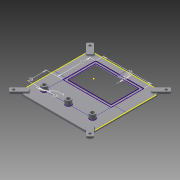
# Autodesk Inventor part: LX4000 2x3slide holder
Saved by Autodesk Inventor 2013 SP2 (Build 170200200, 200)
## iProperties
Created: 2015-05-08
Part Number: LX4000 2x3slide holder
Material: Generic
Document SubType Name: Modeling
Designer: kthorn
Density: 1 g/cm^3
Author: kthorn
Autodesk Inventor part; units mm, degrees
ref_plane "YZ Plane" through (0, 0, 0) normal (1, 0, 0) x (0, 1, 0)
ref_plane "XZ Plane" through (0, 0, 0) normal (0, 1, 0) x (-1, 0, 0)
ref_plane "XY Plane" through (0, 0, 0) normal (0, 0, 1) x (1, 0, 0)
sketch "Sketch1" plane through (0, 0, 0) normal (0, 0, 1) x (1, 0, 0)
  line L0 (-34.939227, 36.850829) -> (65.060773, 36.850829)
  line L1 (73.060773, 28.850829) -> (73.060773, -71.149171)
  line L2 (65.060773, -79.149171) -> (-34.939227, -79.149171)
  line L3 (-42.939227, -71.149171) -> (-42.939227, 28.850829)
  arc A0 (-34.939227, 36.850829) -> (-42.939227, 28.850829) centre (-34.939227, 28.850829) ccw
  arc A1 (-42.939227, -71.149171) -> (-34.939227, -79.149171) centre (-34.939227, -71.149171) ccw
  arc A2 (65.060773, -79.149171) -> (73.060773, -71.149171) centre (65.060773, -71.149171) ccw
  arc A3 (73.060773, 28.850829) -> (65.060773, 36.850829) centre (65.060773, 28.850829) ccw
  point P0 (0, 0)
  point P1 (-42.939227, 36.850829)
  point P2 (73.060773, 36.850829)
  dimension "d0" = 116
  dimension "d2" = 8
  constraints: 8 end point, 8 point on circle, 8 tangent, 4 centre point, 4 point on line, 3 equal radius, 2 parallel, 2 perpendicular, 1 horizontal
  measures "d0" distance of point (-42.939, 36.851) point (73.061, 36.851)
  measures "d2" radius of A0
extrude "Extrusion1" add sketch "Sketch1" along normal blind 3.1
sketch "Sketch2" plane through (0, 0, 3.1) normal (0, 0, 1) x (1, 0, 0)
  line L0 (-42.939227, 28.850829) -> (-42.939227, -71.149171)
  line L1 (73.060773, -71.149171) -> (73.060773, 28.850829)
  line L2 (65.060773, 36.850829) -> (-34.939227, 36.850829)
  line L3 (-23.939227, 26.850829) -> (54.060773, 26.850829)
  line L4 (54.060773, 26.850829) -> (54.060773, -26.149171)
  line L5 (54.060773, -26.149171) -> (-23.939227, -26.149171)
  line L6 (-23.939227, -26.149171) -> (-23.939227, 26.850829)
  line L7 (-19.939227, 22.850829) -> (50.060773, 22.850829)
  line L8 (50.060773, 22.850829) -> (50.060773, -22.149171)
  line L9 (50.060773, -22.149171) -> (-19.939227, -22.149171)
  line L10 (-19.939227, -22.149171) -> (-19.939227, 22.850829)
  line L11 (15.060773, -26.149171) -> (15.060773, -22.149171) construction
  line L12 (-23.939227, 0.350829) -> (-19.939227, 0.350829) construction
  line L13 (15.060773, 26.850829) -> (15.060773, 22.850829) construction
  line L14 (50.060773, 0.350829) -> (54.060773, 0.350829) construction
  line L15 (-23.939227, -21.149171) -> (-42.939227, -21.149171) construction
  line L16 (54.060773, -21.149171) -> (73.060773, -21.149171) construction
  line L17 (15.060773, 36.850829) -> (15.060773, 26.850829) construction
  dimension "d5" = 78
  dimension "d7" = 53
  dimension "d8" = 4
  dimension "d23" = 10
  constraints: 30 end point, 12 midpoint, 8 perpendicular, 4 equal length, 4 parallel, 2 horizontal, 2 point on line, 1 vertical
  measures "d5" distance of L3.start L3.end
  measures "d7" distance of L5.end L3.start
  measures "d8" distance of L13.start L13.end
  measures "d23" distance of L17.start L17.end
extrude "Extrusion2" cut sketch "Sketch2" against normal up to next contours L7 L8 L9 L10
extrude "Extrusion3" cut sketch "Sketch2" against normal blind 1.5
sketch "Sketch3" plane through (0, 0, 3.1) normal (0, 0, 1) x (1, 0, 0)
  line L0 (-34.939227, -79.149171) -> (65.060773, -79.149171)
  line L1 (65.060773, 36.850829) -> (-34.939227, 36.850829)
  line L2 (-42.939227, -71.149171) -> (-42.939227, -79.149171) construction
  line L3 (-34.939227, -79.149171) -> (-42.939227, -79.149171) construction
  line L4 (-42.939227, -79.149171) -> (-42.939227, -82.899171) construction
  line L5 (-42.939227, -82.899171) -> (-46.689227, -82.899171) construction
  line L6 (-32.658004, -75.231909) -> (-46.093032, -88.666938)
  line L7 (-48.92146, -88.666938) -> (-52.456993, -85.131404)
  line L8 (-52.456993, -82.302977) -> (-39.021965, -68.867948)
  line L9 (-36.193538, -68.867948) -> (-32.658004, -72.403482)
  line L10 (-46.689227, -82.899171) -> (-46.689227, -86.899171) construction
  line L11 (-46.689227, -86.899171) -> (-50.689227, -86.899171) construction
  circle A0 centre (-46.689227, -82.899171) radius 2
  arc A1 (-52.456993, -82.302977) -> (-52.456993, -85.131404) centre (-51.04278, -83.71719) ccw
  arc A2 (-48.92146, -88.666938) -> (-46.093032, -88.666938) centre (-47.507246, -87.252724) ccw
  arc A3 (-36.193538, -68.867948) -> (-39.021965, -68.867948) centre (-37.607751, -70.282162) ccw
  arc A4 (-32.658004, -75.231909) -> (-32.658004, -72.403482) centre (-34.072217, -73.817696) ccw
  line L12 (-23.939227, -26.149171) -> (-23.939227, 26.850829)
  line L13 (-23.939227, 26.850829) -> (54.060773, 26.850829)
  line L14 (54.060773, 26.850829) -> (54.060773, -26.149171)
  line L15 (54.060773, -26.149171) -> (-23.939227, -26.149171)
  line L16 (-42.939227, 28.850829) -> (-42.939227, -71.149171)
  arc A5 (-42.939227, -71.149171) -> (-34.939227, -79.149171) centre (-34.939227, -71.149171) ccw
  line L17 (-34.939227, -79.149171) -> (65.060773, -79.149171)
  arc A6 (65.060773, -79.149171) -> (73.060773, -71.149171) centre (65.060773, -71.149171) ccw
  line L18 (73.060773, -71.149171) -> (73.060773, 28.850829)
  arc A7 (73.060773, 28.850829) -> (65.060773, 36.850829) centre (65.060773, 28.850829) ccw
  line L19 (65.060773, 36.850829) -> (-34.939227, 36.850829)
  arc A8 (-34.939227, 36.850829) -> (-42.939227, 28.850829) centre (-34.939227, 28.850829) ccw
  line L20 (15.060773, -79.149171) -> (15.060773, 36.850829) construction
  line L21 (73.060773, -21.149171) -> (-42.939227, -21.149171) construction
  line L22 (73.060773, -71.149171) -> (73.060773, -79.149171) construction
  line L23 (65.060773, -79.149171) -> (73.060773, -79.149171) construction
  line L24 (73.060773, -79.149171) -> (73.060773, -82.899171) construction
  line L25 (73.060773, -82.899171) -> (76.810773, -82.899171) construction
  line L26 (62.779551, -75.231909) -> (76.214579, -88.666938)
  line L27 (79.043007, -88.666938) -> (82.57854, -85.131404)
  line L28 (82.57854, -82.302977) -> (69.143512, -68.867948)
  line L29 (66.315084, -68.867948) -> (62.779551, -72.403482)
  line L30 (76.810773, -82.899171) -> (76.810773, -86.899171) construction
  line L31 (76.810773, -86.899171) -> (80.810773, -86.899171) construction
  circle A9 centre (76.810773, -82.899171) radius 2
  arc A10 (82.57854, -85.131404) -> (82.57854, -82.302977) centre (81.164327, -83.71719) ccw
  arc A11 (76.214579, -88.666938) -> (79.043007, -88.666938) centre (77.628793, -87.252724) ccw
  arc A12 (69.143512, -68.867948) -> (66.315084, -68.867948) centre (67.729298, -70.282162) ccw
  arc A13 (62.779551, -72.403482) -> (62.779551, -75.231909) centre (64.193764, -73.817696) ccw
  arc A14 (65.060773, -79.149171) -> (73.060773, -71.149171) centre (65.060773, -71.149171) ccw
  line L32 (-42.939227, 28.850829) -> (-42.939227, 36.850829) construction
  line L33 (-34.939227, 36.850829) -> (-42.939227, 36.850829) construction
  line L34 (-42.939227, 36.850829) -> (-42.939227, 40.600829) construction
  line L35 (-42.939227, 40.600829) -> (-46.689227, 40.600829) construction
  line L36 (-32.658004, 32.933567) -> (-46.093032, 46.368596)
  line L37 (-48.92146, 46.368596) -> (-52.456993, 42.833062)
  line L38 (-52.456993, 40.004635) -> (-39.021965, 26.569606)
  line L39 (-36.193538, 26.569606) -> (-32.658004, 30.10514)
  line L40 (-46.689227, 40.600829) -> (-46.689227, 44.600829) construction
  line L41 (-46.689227, 44.600829) -> (-50.689227, 44.600829) construction
  circle A15 centre (-46.689227, 40.600829) radius 2
  arc A16 (-52.456993, 42.833062) -> (-52.456993, 40.004635) centre (-51.04278, 41.418849) ccw
  arc A17 (-46.093032, 46.368596) -> (-48.92146, 46.368596) centre (-47.507246, 44.954382) ccw
  arc A18 (-39.021965, 26.569606) -> (-36.193538, 26.569606) centre (-37.607751, 27.98382) ccw
  arc A19 (-32.658004, 30.10514) -> (-32.658004, 32.933567) centre (-34.072217, 31.519354) ccw
  arc A20 (-34.939227, 36.850829) -> (-42.939227, 28.850829) centre (-34.939227, 28.850829) ccw
  arc A21 (73.060773, 28.850829) -> (65.060773, 36.850829) centre (65.060773, 28.850829) ccw
  arc A22 (62.779551, 32.933567) -> (62.779551, 30.10514) centre (64.193764, 31.519354) ccw
  line L42 (66.315084, 26.569606) -> (62.779551, 30.10514)
  arc A23 (66.315084, 26.569606) -> (69.143512, 26.569606) centre (67.729298, 27.98382) ccw
  arc A24 (73.060773, 28.850829) -> (65.060773, 36.850829) centre (65.060773, 28.850829) ccw
  line L43 (73.060773, 28.850829) -> (73.060773, 36.850829) construction
  line L44 (65.060773, 36.850829) -> (73.060773, 36.850829) construction
  line L45 (73.060773, 36.850829) -> (73.060773, 40.600829) construction
  line L46 (73.060773, 40.600829) -> (76.810773, 40.600829) construction
  line L47 (62.779551, 32.933567) -> (76.214579, 46.368596)
  line L48 (79.043007, 46.368596) -> (82.57854, 42.833062)
  line L49 (82.57854, 40.004635) -> (69.143512, 26.569606)
  line L50 (76.810773, 40.600829) -> (76.810773, 44.600829) construction
  line L51 (76.810773, 44.600829) -> (80.810773, 44.600829) construction
  circle A25 centre (76.810773, 40.600829) radius 2
  arc A26 (82.57854, 40.004635) -> (82.57854, 42.833062) centre (81.164327, 41.418849) ccw
  arc A27 (79.043007, 46.368596) -> (76.214579, 46.368596) centre (77.628793, 44.954382) ccw
  arc A28 (-42.939227, -71.149171) -> (-34.939227, -79.149171) centre (-34.939227, -71.149171) ccw
  line L52 (-34.939227, -71.149171) -> (-42.939227, -79.149171) construction
  point P0 (0, 0)
  point P1 (-31.24379, -73.817696)
  point P2 (-37.607751, -67.453734)
  point P3 (-34.425771, -70.635715)
  point P4 (61.365337, -73.817696)
  point P5 (67.729298, -67.453734)
  point P6 (64.547318, -70.635715)
  point P7 (-31.24379, 31.519354)
  point P8 (-37.607751, 25.155393)
  point P9 (-34.425771, 28.337373)
  point P10 (61.365337, 31.519354)
  point P11 (67.729298, 25.155393)
  point P12 (64.547318, 28.337373)
  dimension "d13" = 3.75
  dimension "d15" = 4
  dimension "d16" = 4
  dimension "d17" = 9
  dimension "d18" = 2
  dimension "d32" = 23
  constraints: 86 end point, 83 symmetric about line, 40 point on circle, 24 centre point, 16 point on line, 10 perpendicular, 8 tangent, 6 midpoint, 4 coincident, 3 equal radius, 2 parallel, 19 other
  measures "d13" distance of L4.end L5.end
  measures "d15" distance of L11.end L10.end
  measures "d16" diameter of A0
  measures "d17" distance of point (-37.608, -67.454) point (-31.244, -73.818)
  measures "d18" radius of A1
  measures "d32" distance between parallel lines of L7 L9
extrude "Extrusion4" add sketch "Sketch3" along normal blind 3 contours A5 L8 A3 L9 A4 L6 | L6 A2 L7 A1 L8 A5 | L26 A13 L29 A12 L28 A6 | A6 L28 A10 L27 A11 L26 | L38 A16 L37 A17 L36 A8 | A8 L36 A19 L39 A18 L38 | L49 A23 L42 A22 L47 A7 | A7 L47 A27 L48 A26 L49
fillet "Fillet1" radius 2 5 edges at (62.1938, -73.8177, 3.1) (64.5473, -70.6357, 3.1) (67.7293, -68.2822, 3.1) (71.0317, -70.7561, 3.1) (64.6677, -77.1201, 3.1)
fillet "Fillet2" radius 2 15 edges at (-32.0722, -73.8177, 3.1) (-34.4258, -70.6357, 3.1) (-37.6078, -68.2822, 3.1) (-40.9101, -70.7561, 3.1) (-34.5462, -77.1201, 3.1) (64.5473, 28.3374, 3.1) (62.1938, 31.5194, 3.1) (64.6677, 34.8217, 3.1) (71.0317, 28.4578, 3.1) (67.7293, 25.9838, 3.1) (-40.9101, 28.4578, 3.1) (-34.4258, 28.3374, 3.1) (-32.0722, 31.5194, 3.1) (-34.5462, 34.8217, 3.1) (-37.6078, 25.9838, 3.1)
sketch "Sketch4" plane through (0, 0, 3.1) normal (0, 0, 1) x (1, 0, 0)
  line L0 (54.060773, -26.149171) -> (-23.939227, -26.149171)
  line L1 (-23.939227, -26.149171) -> (-23.939227, -56.149171) construction
  line L2 (54.060773, -26.149171) -> (54.060773, -56.149171) construction
  circle A0 centre (-23.939227, -56.149171) radius 2.8
  circle A1 centre (54.060773, -56.149171) radius 2.8
  circle A2 centre (-23.939227, -56.149171) radius 4.5
  circle A3 centre (54.060773, -56.149171) radius 4.5
  line L3 (-23.939227, -56.149171) -> (54.060773, -56.149171) construction
  circle A4 centre (15.060773, -56.149171) radius 4.5
  circle A5 centre (15.060773, -56.149171) radius 2.8
  point P0 (0, 0)
  dimension "d24" = 30
  dimension "d25" = 5.6
  dimension "d26" = 9
  constraints: 6 centre point, 6 end point, 5 coincident, 4 equal radius, 2 parallel, 2 perpendicular, 1 midpoint
  measures "d24" distance of L0.end L1.end
  measures "d25" diameter of A0
  measures "d26" diameter of A2
extrude "Extrusion5" add sketch "Sketch4" along normal blind 7.8
extrude "Extrusion6" cut sketch "Sketch4" against normal up to next contours A0 | A1 | A5
body "Solid1"
